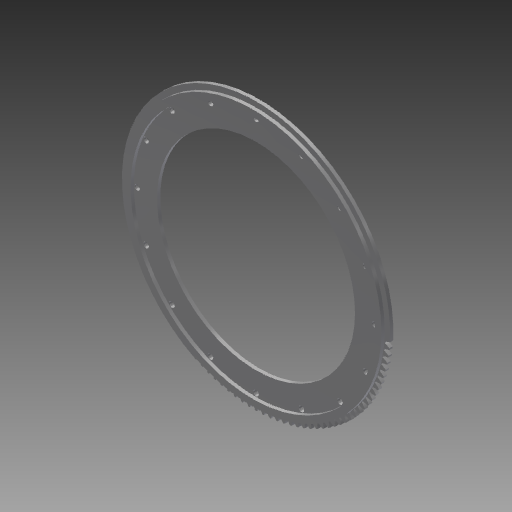
# Autodesk Inventor part: Spur Gear2
Saved by Autodesk Inventor 2019 (Build 230136000, 136)
## iProperties
Created: 2020-06-08
Part Number: Spur Gear2
Material: Steel
Document SubType Name: Modeling
Designer: Hugo Albarracin
Categories: <?xml version="1.0" encoding="UTF-16"?> <MemberInstance><Categories><FamilyTemplate><FamilyTemplateParameter ValueType="xs:double" Id="1" ObjectReferenceKey="da_z" ObjectType="kUserParameterObject"/><FamilyTemplateParameter ValueType="xs:double" Id="2" ObjectReferenceKey="da_b" ObjectType="kUserParameterObject"/><FamilyTemplateParameter ValueType="xs:double" Id="3" ObjectReferenceKey="da_beta" ObjectType="kUserParameterObject"/><FamilyTemplateParameter ValueType="xs:double" Id="4" ObjectReferenceKey="da_da" ObjectType="kUserParameterObject"/><FamilyTemplateParameter ValueType="xs:double" Id="5" ObjectReferenceKey="da_aw" ObjectType="kUserParameterObject"/><FamilyTemplateParameter ValueType="xs:string" Id="6" ObjectReferenceKey="EAIAABAAAACIAQAAAAAAAIAAAAAAAAAA" ObjectType="83910656" SubObjectId="SurfaceGeometry"/></FamilyTemplate><ParamToTemplateMap><ParamToTemplate CategoryParameter="//CategoryParameter[@InternalName='046C89C9-8512-4d59-83FE-43B91F4F132A']" TemplateParameter="1"/><ParamToTemplate CategoryParameter="//CategoryParameter[@InternalName='2552DF32-E462-4b46-AEBF-C6C7768E72AC']" TemplateParameter="2"/><ParamToTemplate CategoryParameter="//CategoryParameter[@InternalName='C9EE641D-15FC-4fae-A226-E94C4372FDD7']" TemplateParameter="3"/><ParamToTemplate><ParamToTemplate CategoryParameter="//CategoryParameter[@InternalName='00B6519A-459B-49c7-AD84-2E56D39A5744']" ConstantValue="-0.050502"/></ParamToTemplate><ParamToTemplate><ParamToTemplate CategoryParameter="//CategoryParameter[@InternalName='04B31F0E-C7A6-4894-AA32-9629BEFACF47']" ConstantValue="1.000000"/></ParamToTemplate><ParamToTemplate><ParamToTemplate CategoryParameter="//CategoryParameter[@InternalName='43CBEC2E-7847-49e7-A936-2F7889FCB2D9']" ConstantValue="0.250000"/></ParamToTemplate><ParamToTemplate><ParamToTemplate CategoryParameter="//CategoryParameter[@InternalName='B1EFC894-105D-4ebd-86BF-FA20ED196853']" ConstantValue="0.350000"/></ParamToTemplate><ParamToTemplate><ParamToTemplate CategoryParameter="//CategoryParameter[@InternalName='51175063-3D10-4879-93E8-6246FE8B403D']" ConstantValue="2060000000.000000"/></ParamToTemplate><ParamToTemplate><ParamToTemplate CategoryParameter="//CategoryParameter[@InternalName='A3A52E27-4454-46a9-B0BD-C932399B70AF']" ConstantValue="0.300000"/></ParamToTemplate><ParamToTemplate><ParamToTemplate CategoryParameter="//CategoryParameter[@InternalName='91B76062-C214-41d9-B1B9-14D2AB99603D']" ConstantValue="0.200000"/></ParamToTemplate><ParamToTemplate><ParamToTemplate CategoryParameter="//CategoryParameter[@InternalName='374E806E-8B8A-4dda-A9AA-1039D6500AD2']" ConstantValue="5.000000"/></ParamToTemplate><ParamToTemplate><ParamToTemplate CategoryParameter="//CategoryParameter[@InternalName='2D373A89-B862-43d6-8D0B-0CBF12AB9F6C']" ConstantValue="0.349066"/></ParamToTemplate><ParamToTemplate CategoryParameter="//CategoryParameter[@InternalName='37777632-D6A2-4fac-9D53-DB8ACD95C989']" TemplateParameter="4"/><ParamToTemplate CategoryParameter="//CategoryParameter[@InternalName='FD1017F1-B727-4f7e-9707-0F86F1FF9423']" TemplateParameter="5"/><ParamToTemplate><ParamToTemplate CategoryParameter="//CategoryParameter[@InternalName='9E1B4470-B2D3-4ff1-B813-535BB4CDF51A']" ConstantValue="3520000.000000"/></ParamToTemplate><ParamToTemplate><ParamToTemplate CategoryParameter="//CategoryParameter[@InternalName='F8452263-BFF6-458c-9FB1-07C4B99E95CD']" ConstantValue="11400000.000000"/></ParamToTemplate><ParamToTemplate><ParamToTemplate CategoryParameter="//CategoryParameter[@InternalName='3E3BB259-FD49-497f-8171-6EBC954A3479']" ConstantValue="2.000000"/></ParamToTemplate><ParamToTemplate CategoryParameter="//CategoryParameter[@InternalName='27C3BAF2-7550-4e4b-AE2C-0DB134B7D9B7']" TemplateParameter="6"/></ParamToTemplateMap><Category DisplayName="Gear" InternalName="DC85795E-93AB-48d5-8EEE-5A27447B64BD" Mnemonic="Gear"><CategoryParameter DisplayName="z" InternalName="046C89C9-8512-4d59-83FE-43B91F4F132A" Mnemonic="z"/><CategoryParameter DisplayName="b" InternalName="2552DF32-E462-4b46-AEBF-C6C7768E72AC" Mnemonic="b"/><CategoryParameter DisplayName="||b|" InternalName="C9EE641D-15FC-4fae-A226-E94C4372FDD7" Mnemonic="beta"/><CategoryParameter DisplayName="x" InternalName="00B6519A-459B-49c7-AD84-2E56D39A5744" Mnemonic="x"/><CategoryParameter DisplayName="a*" InternalName="04B31F0E-C7A6-4894-AA32-9629BEFACF47" Mnemonic="a"/><CategoryParameter DisplayName="c*" InternalName="43CBEC2E-7847-49e7-A936-2F7889FCB2D9" Mnemonic="c"/><CategoryParameter DisplayName="r|.f|*" InternalName="B1EFC894-105D-4ebd-86BF-FA20ED196853" Mnemonic="rf"/><CategoryParameter DisplayName="E" InternalName="51175063-3D10-4879-93E8-6246FE8B403D" Mnemonic="E"/><CategoryParameter DisplayName="||m|" InternalName="A3A52E27-4454-46a9-B0BD-C932399B70AF" Mnemonic="mi"/><Category DisplayName="SpurGear" InternalName="26C5A22E-A91E-4dfd-A3B3-23CCAFAE1764" Mnemonic="SpurGear"><CategoryParameter DisplayName="m" InternalName="91B76062-C214-41d9-B1B9-14D2AB99603D" Mnemonic="m"/><CategoryParameter DisplayName="P" InternalName="374E806E-8B8A-4dda-A9AA-1039D6500AD2" Mnemonic="PP"/><CategoryParameter DisplayName="||a|" InternalName="2D373A89-B862-43d6-8D0B-0CBF12AB9F6C" Mnemonic="alpha"/><CategoryParameter DisplayName="d|.a|" InternalName="37777632-D6A2-4fac-9D53-DB8ACD95C989" Mnemonic="da"/><CategoryParameter DisplayName="a|.w|" InternalName="FD1017F1-B727-4f7e-9707-0F86F1FF9423" Mnemonic="aw"/><CategoryParameter DisplayName="||s||.Flim|" InternalName="9E1B4470-B2D3-4ff1-B813-535BB4CDF51A" Mnemonic="sFlim"/><CategoryParameter DisplayName="||s||.Hlim|" InternalName="F8452263-BFF6-458c-9FB1-07C4B99E95CD" Mnemonic="sHlim"/><CategoryParameter DisplayName="type" InternalName="3E3BB259-FD49-497f-8171-6EBC954A3479" Mnemonic="type"/><CategoryParameter DisplayName="PitchDiameter" InternalName="27C3BAF2-7550-4e4b-AE2C-0DB134B7D9B7" Mnemonic="IDS_PITCHDIAM"/></Category></Category></Categories></MemberInstance>
Density: 1 g/cm^3
Appearance: Steel
CustomPartVersion: 1
Author: Hugo Albarracin
Autodesk Inventor part; units mm, degrees
sketch "Sketch1" plane through (0, 0, 0) normal (0, 0, 1) x (1, 0, 0)
  circle A0 centre (0, 0) radius 121.85
  dimension "d0" = 243.7
  constraints: 1 centre point
  measures "d0" diameter of A0
extrude "Extrusion1" add sketch "Sketch1" along normal blind 3
ref_plane "Work Plane2" through (0, 0, 1.5) normal (0, 0, 1) x (1, 0, 0)
sketch "Sketch2" plane through (0, 0, 0) normal (0, 0, -1) x (-1, 0, 0)
  circle A0 centre (0, 0) radius 121.85 projected
  circle A1 centre (0, 0) radius 100
  dimension "d3" = 200
  constraints: 1 centre point, 1 coincident
  measures "d3" diameter of A1
surface extrude "Pitch Diameter" sketch "Sketch2" against normal through all shown no curves A1
ref_plane "Work Plane8" through (0, 0, 0) normal (0.9996573, 0.0261769, 0) x (0, 0, 1)
ref_plane "Work Plane9" through (0, 0, 0) normal (1, 0, 0) x (0, 1, 0)
spur gear teeth "Spur Gear" teeth 120 pitch diameter 240 tip diameter 243.7 root diameter 234.7 face width 3 start plane through (0, 0, 0) normal (0, 0, -1) x (-1, 0, 0)
sketch "Sketch3" plane through (0, 0, 3) normal (0, 0, 1) x (1, 0, 0)
  circle A0 centre (0, 0) radius 90
  dimension "d49" = 180
  constraints: 1 centre point, 1 coincident
  measures "d49" diameter of A0
extrude "Extrusion2" cut sketch "Sketch3" against normal blind 10
sketch "Sketch4" plane through (0, 0, 3) normal (0, 0, 1) x (1, 0, 0)
  circle A0 centre (108, 0) radius 2.5
  line L0 (0, 0) -> (108, 0) construction
  circle A1 centre (0, 0) radius 90 construction
  circle A2 centre (0, 0) radius 108 construction
  dimension "d52" = 5
  dimension "d102" = 18
  constraints: 2 end point, 1 centre point, 1 coincident, 1 horizontal, 1 horizontal alignment, 2 other
  measures "d52" diameter of A0
extrude "Extrusion3" cut sketch "Sketch4" against normal blind 10
sketch "Sketch5" plane through (0, 0, 3) normal (0, 0, 1) x (1, 0, 0)
  circle A0 centre (0, 0) radius 121.85 projected
  line L0 (-52.1868, -102.4223) -> (-55.3187, -108.5691)
  arc A1 (121.683, -6.3771) -> (-55.3187, -108.5691) centre (0, 0) ccw
  arc A2 (114.7937, -6.0161) -> (-52.1868, -102.4223) centre (0, 0) ccw
  line L1 (-52.1868, -102.4223) -> (0, 0) construction
  line L2 (0, 0) -> (114.9513, 0) construction
  line L3 (114.7937, -6.0161) -> (121.683, -6.3771)
  line L4 (0, 0) -> (114.7937, -6.0161) construction
  point P0 (121.85, 0)
  point P1 (121.8474, 0.7975)
  point P2 (121.8474, -0.7975)
  point P3 (0.7975, 121.8474)
  point P4 (-0.7975, 121.8474)
  dimension "d63" = 3
  dimension "d64" = 114
  dimension "d103" = 6.8987
  constraints: 10 end point, 7 point on circle, 2 centre point, 2 coincident, 2 collinear, 1 horizontal
  measures "d63" angle of L2 L4
  measures "d64" angle of L1 L4
  measures "d103" radial gap between concentric circles of A2 A1
extrude "Extrusion4" add sketch "Sketch5" against normal blind 3 contours A0 L3 A2 L0 picked at (-107.987, 45.2611)
sketch "Sketch6" plane through (0, 0, 3) normal (0, 0, 1) x (1, 0, 0)
  circle A0 centre (0, 0) radius 90 projected
  line L0 (0, 0) -> (-90, 0) construction
  line L1 (0, 0) -> (-50.0013, -74.8323)
  line L2 (-58.8904, -88.1358) -> (-63.0478, -85.3579) construction
  line L3 (-63.0478, -85.3579) -> (-58.6032, -78.7062)
  line L4 (-63.0478, -85.3579) -> (-67.4924, -92.0097)
  line L5 (-67.4924, -92.0097) -> (-65.8294, -93.1208)
  line L6 (-58.6032, -78.7062) -> (-56.9403, -79.8173)
  line L7 (-56.9403, -79.8173) -> (-56.6682, -84.8099)
  line L8 (-65.8294, -93.1208) -> (-61.1127, -91.4617)
  line L9 (-50.0013, -74.8323) -> (-56.6682, -84.8099)
  line L10 (-61.1127, -91.4617) -> (-67.7796, -101.4393)
  line L11 (-58.8904, 88.1358) -> (-54.7331, 90.9136) construction
  line L12 (-54.7331, 90.9136) -> (-50.2885, 84.2619)
  line L13 (-54.7331, 90.9136) -> (-59.1777, 97.5654)
  line L14 (-59.1777, 97.5654) -> (-60.8406, 96.4542)
  line L15 (-50.2885, 84.2619) -> (-51.9515, 83.1507)
  line L16 (-51.9515, 83.1507) -> (-56.6682, 84.8099)
  line L17 (-60.8406, 96.4542) -> (-61.1127, 91.4617)
  line L18 (-50.0013, 74.8323) -> (-56.6682, 84.8099)
  line L19 (-61.1127, 91.4617) -> (-67.7796, 101.4393)
  line L20 (97.0924, 14.2149) -> (96.7022, 16.1765)
  line L21 (96.7022, 16.1765) -> (100.0401, 19.8992)
  line L22 (88.2707, 17.5581) -> (100.0401, 19.8992)
  line L23 (104.9387, 15.7756) -> (97.0924, 14.2149)
  line L24 (103.9632, 20.6796) -> (104.9387, 15.7756) construction
  line L25 (112.3948, 19.2979) -> (107.8864, 21.4599)
  line L26 (104.9387, 15.7756) -> (112.785, 17.3364)
  line L27 (112.785, 17.3364) -> (112.3948, 19.2979)
  line L28 (107.8864, 21.4599) -> (119.6558, 23.801)
  line L29 (0, 0) -> (-50.0013, 74.8323)
  line L30 (0, 0) -> (88.2707, 17.5581)
  dimension "d65" = 122
  dimension "d68" = 56.25
  dimension "d69" = 5
  dimension "d70" = 8
  dimension "d71" = 8
  dimension "d72" = 2
  dimension "d73" = 4
  dimension "d74" = 4
  dimension "d75" = 5
  dimension "d76" = 8
  dimension "d77" = 8
  dimension "d78" = 2
  dimension "d79" = 4
  dimension "d80" = 4
  dimension "d81" = 5
  dimension "d82" = 8
  dimension "d83" = 8
  dimension "d84" = 2
  dimension "d85" = 4
  dimension "d86" = 4
  dimension "d89" = 112.5
  dimension "d90" = 112.5
  dimension "d91" = 5
  dimension "d92" = 5
  dimension "d93" = 16
  dimension "d94" = 16
  constraints: 62 end point, 6 perpendicular, 5 collinear, 3 parallel, 3 point on line, 2 point on circle, 1 horizontal
  measures "d65" distance of point (0, 0) L10.end
  measures "d68" angle of L1 L0
  measures "d69" distance of L2.start L2.end
  measures "d70" distance of L2.end L3.end
  measures "d71" distance of L2.end L4.end
  measures "d72" distance of L4.end L5.end
  measures "d73" distance from line of L8.end L2
  measures "d74" distance from line of L7.end L2
  measures "d75" distance of L11.start L12.start
  measures "d76" distance of L12.start L15.start
  measures "d77" distance of L12.start L13.end
  measures "d78" distance of L13.end L17.start
  measures "d79" distance from line of L17.end L11
  measures "d80" distance from line of L16.end L11
  measures "d81" distance of L24.start L23.start
  measures "d82" distance of L23.start L20.start
  measures "d83" distance of L23.start L27.start
  measures "d84" distance of L27.start L25.start
  measures "d85" distance from line of L25.end L24
  measures "d86" distance from line of L22.end L24
  measures "d89" angle of L29 L1
  measures "d90" angle of L30 L29
  measures "d91" distance between parallel lines of L12 L18
  measures "d92" distance between parallel lines of L22 L23
  measures "d93" distance from line of L22.start L24
  measures "d94" distance from line of L18.start L11
sketch "Sketch7" plane through (0, 0, 3) normal (0, 0, 1) x (1, 0, 0)
  circle A0 centre (0, 0) radius 117
  circle A1 centre (0, 0) radius 111
  dimension "d95" = 234
  dimension "d96" = 6
  constraints: 2 centre point, 1 coincident
  measures "d95" diameter of A0
  measures "d96" radial gap between concentric circles of A0 A1
extrude "Extrusion5" add sketch "Sketch7" along normal blind 3
pattern_circular "Circular Pattern2" count 16 over 360 about axis through (0, 0, 3) along (0, 0, -1) of "Extrusion3"
equation "\"d0\" = da_da"
equation "\"d1\" = da_b"
equation "\"da_d\" = da_dw"
equation "\"da_aw\" = 2 * num_z"
equation "\"da_dw\" = 2 * num_z"
equation "\"d49\" = diametro_max - 2 * ancho_disco"
equation "\"angulo_alabe\" = 130deg"
equation "\"diametro_tubo\" = 232"
equation "\"desfase_a_pin_superior\" = 12"
equation "\"desfase_b_pin_inferior\" = 8"
equation "\"desfase_b_pin_superior\" = 0"
equation "\"diametro_max_soporte\" = 248"
equation "\"da_da\" = 243.7"
equation "\"da_b\" = 3"
equation "\"num_z\" = 120"
equation "\"diametro_max\" = 240"
equation "\"ancho_disco\" = 30"
body "Solid1"
body "Srf1"
